pin (Autodesk Fusion 360 design; units mm, degrees)
part number: 2026-09-20-22-03-39-965
Autodesk Fusion 360 part; units mm, degrees
sketch "Sketch2" plane through (0, 0, 0) normal (0, 0, 1) x (1, 0, 0)
  circle A0 centre (-26, 11) radius 2
  dimension "d5" = 4
  measures "d5" diameter of A0
extrude "Extrude2" add sketch "Sketch2" along normal blind 22
chamfer "Chamfer2" distance 0.15 angle 45 1 faces at (-24.0025, 10.9003, 14.6667)
sketch "Sketch1" plane through (0, 0, 0) normal (0, 0, 1) x (1, 0, 0)
  circle A0 centre (-66, 26) radius 1.5
  dimension "d1" = 3
  measures "d1" diameter of A0
extrude "Extrude1" [suppressed]
chamfer "Chamfer1" [suppressed]
